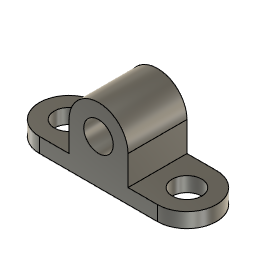
A4 (Autodesk Fusion 360 design; units mm, degrees)
Autodesk Fusion 360 part; units mm, degrees
sketch "Sketch1" plane through (0, 0, 0) normal (0, 0, 1) x (1, 0, 0)
  line L0 (20, 19) -> (100, 19)
  line L1 (120, -1) -> (120, -1)
  line L2 (100, -21) -> (20, -21)
  line L3 (0, -1) -> (0, -1)
  line L4 (20.2852, -21) -> (100.2852, -21)
  line L5 (20, 19) -> (100, 19)
  arc A0 (20, 19) -> (0, -1) centre (20, -1) ccw
  arc A1 (0, -1) -> (20, -21) centre (20, -1) ccw
  arc A2 (120, -1) -> (100, 19) centre (100, -1) ccw
  arc A3 (100, -21) -> (120, -1) centre (100, -1) ccw
  circle A4 centre (20, -1.0086) radius 10
  circle A5 centre (100, -1) radius 10
  point P0 (0, 19)
  point P1 (120, 19)
  point P2 (0, -21)
  dimension "d1" = 120
  dimension "d2" = 40
  dimension "d5" = 20
  dimension "d6" = 20
  dimension "d7" = 20
  dimension "d8" = 20
  dimension "d9" = 20
  dimension "d10" = 20
  constraint horizontal L0
  constraint horizontal L2
  constraint coincident L2 L4.start
  constraint coincident L0 L5.start
  constraint coincident L0 L5.end
  constraint coincident P0 L0
  constraint tangent L0 A0
  constraint coincident P2 L2
  constraint coincident P2 L3
  constraint tangent L2 A1
  constraint coincident P1 L0
  constraint tangent L0 A2
  constraint tangent L2 A3
  measures "d1" distance of P0 P1
  measures "d2" distance of P0 P2
  measures "d5" radius of A0
  measures "d6" radius of A1
  measures "d7" radius of A2
  measures "d8" radius of A3
  measures "d9" diameter of A4
  measures "d10" diameter of A5
extrude "Extrude1" add sketch "Sketch1" along normal blind 10
sketch "Sketch2" plane through (0, 0, 10) normal (0, 0, 1) x (-1, 0, 0)
  circle A0 centre (-100, 1) radius 10
  circle A1 centre (-20, 1.0086) radius 10
  line L0 (-20, 21) -> (-100, 21)
  arc A2 (-100, 21) -> (-100, -19) centre (-100, 1) ccw
  line L1 (-100, -19) -> (-20, -19)
  arc A3 (-20, -19) -> (-20, 21) centre (-20, 1) ccw
  line L2 (-40, -19) -> (-80, -19)
  line L3 (-80, -19) -> (-80, 21)
  line L4 (-80, 21) -> (-40, 21)
  line L5 (-40, 21) -> (-40, -19)
  dimension "d13" = 40
  constraint horizontal L2
  constraint vertical L3
  constraint horizontal L4
  constraint vertical L5
  constraint coincident L1 L2.start
  measures "d13" distance of L2.start L2.end
extrude "Extrude2" add sketch "Sketch2" along normal blind 40 contours L0 L1 L2 L3 L4 L5
fillet "Fillet1" radius 20 2 edges at (40, -1, 50) (80, -1, 50)
sketch "Sketch3" plane through (0, -21, 0) normal (0, -1, 0) x (1, 0, 0)
  arc A0 (80, 30) -> (40, 30) centre (60, 30) ccw
  line L0 (40, 30) -> (40, 10)
  line L1 (40, 10) -> (20, 10)
  line L2 (20, 10) -> (20, 0)
  line L3 (20, 0) -> (100, 0)
  line L4 (100, 0) -> (100, 10)
  line L5 (100, 10) -> (80, 10)
  line L6 (80, 10) -> (80, 30)
  circle A1 centre (60, 30) radius 10
  dimension "d18" = 20
  constraint concentric A0 A1
  measures "d18" diameter of A1
extrude "Extrude3" cut sketch "Sketch3" against normal blind 40 contours A1
named bodies: "A4"
